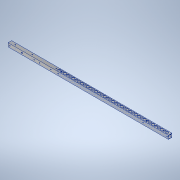
# Autodesk Inventor part: ロボットベース15x15_3
Saved by Autodesk Inventor 2020.3 (Build 243373000, 373)
## iProperties
Created: 2020-07-04
Part Number: ロボットベース15x15_3
Material: アルミニウム 6061
Document SubType Name: Modeling
Designer: totot
Density: 2.7 g/cm^3
Appearance: アルミニウム - フラット
Mass: 98.5001 g
Surface Area: 641.394 cm^2
Volume: 36.4815 cm^3
Author: totot
Autodesk Inventor part; units mm, degrees
ref_plane "YZ Plane" through (0, 0, 0) normal (1, 0, 0) x (0, 1, 0)
ref_plane "XZ Plane" through (0, 0, 0) normal (0, 1, 0) x (-1, 0, 0)
ref_plane "XY Plane" through (0, 0, 0) normal (0, 0, 1) x (1, 0, 0)
sketch "スケッチ1" plane through (0, 0, 0) normal (1, 0, 0) x (0, 1, 0)
  line L0 (0, 0) -> (-15, 0)
  line L1 (-15, 0) -> (-15, 15)
  line L2 (-15, 15) -> (0, 15)
  line L3 (0, 15) -> (0, 0)
  line L4 (-1.2, 13.8) -> (-13.8, 13.8)
  line L5 (-13.8, 13.8) -> (-13.8, 1.2)
  line L6 (-13.8, 1.2) -> (-1.2, 1.2)
  line L7 (-1.2, 1.2) -> (-1.2, 13.8)
  dimension "d0" = 15
  dimension "d1" = 15
  dimension "d2" = 1.2
  dimension "d3" = 1.2
  dimension "d4" = 1.2
  dimension "d5" = 1.2
  constraints: 16 end point, 4 parallel, 2 horizontal, 2 perpendicular
  measures "d0" distance of L1.end L2.end
  measures "d1" distance of L0.end L1.end
  measures "d2" distance between parallel lines of L2 L4
  measures "d3" distance between parallel lines of L7 L3
  measures "d4" distance between parallel lines of L1 L5
  measures "d5" distance between parallel lines of L0 L6
extrude "押し出し1" add sketch "スケッチ1" along normal blind 116
sketch "スケッチ2" plane through (0, -15, 15) normal (0, 0, 1) x (1, 0, 0)
  line L0 (0, 15) -> (116, 15) projected
  line L1 (0, 15) -> (0, 0) projected
  line L2 (116, 15) -> (116, 0) projected
  point P0 (7.5, 7.5)
  point P1 (108.5, 7.5)
  dimension "d8" = 7.5
  dimension "d9" = 7.5
  dimension "d10" = 7.5
  dimension "d11" = 7.5
  measures "d8" distance from line of L0 point (7.5, 7.5)
  measures "d9" distance from line of point (108.5, 7.5) L0
  measures "d10" distance from line of point (7.5, 7.5) L1
  measures "d11" distance from line of point (108.5, 7.5) L2
hole "穴1" at (7.5, -7.5, 15) at (108.5, -7.5, 15) direction (0, 0, -1) diameter 3 end through all
sketch "スケッチ3" plane through (0, -15, 0) normal (0, 0, -1) x (-1, 0, 0)
  circle A0 centre (-7.5, 7.5) radius 1.5 projected
  line L0 (0, 0) -> (-116, 0) projected
  point P0 (0, 15)
  point P1 (-58, 7.5)
  dimension "d19" = 50.5
  dimension "d20" = 7.5
  measures "d19" distance of point (-58, 7.5) A0.centre
  measures "d20" distance from line of point (-58, 7.5) L0
hole "穴2" at (58, -7.5, 0) direction (0, 0, 1) diameter 5 end through all
sketch "スケッチ4" plane through (0, -15, 0) normal (0, -1, 0) x (1, 0, 0)
  line L0 (0, 15) -> (0, 0) projected
  line L1 (0, 0) -> (116, 0) projected
  line L2 (116, 15) -> (116, 0) projected
  point P0 (22.5, 7.5)
  point P1 (93.5, 7.5)
  dimension "d28" = 22.5
  dimension "d29" = 7.5
  dimension "d30" = 7.5
  dimension "d31" = 22.5
  measures "d28" distance from line of point (22.5, 7.5) L0
  measures "d29" distance from line of point (22.5, 7.5) L1
  measures "d30" distance from line of L1 point (93.5, 7.5)
  measures "d31" distance from line of point (93.5, 7.5) L2
hole "穴3" at (22.5, -15, 7.5) at (93.5, -15, 7.5) direction (0, 1, 0) diameter 3 end through all
sketch "スケッチ5" plane through (116, 0, 0) normal (1, 0, 0) x (0, 0, -1)
  line L0 (0, 0) -> (-15, 0)
  line L1 (-15, 0) -> (-15, -15)
  line L2 (-15, -15) -> (0, -15)
  line L3 (0, -15) -> (0, 0)
  line L4 (-13.8, -1.2) -> (-1.2, -1.2) projected
  line L5 (-1.2, -1.2) -> (-13.8, -1.2)
  line L6 (-13.8, -1.2) -> (-13.8, -13.8)
  line L7 (-13.8, -13.8) -> (-1.2, -13.8)
  line L8 (-1.2, -13.8) -> (-1.2, -1.2)
  dimension "d39" = 15
  dimension "d40" = 15
  constraints: 16 end point, 4 parallel, 2 horizontal, 2 perpendicular
  measures "d39" distance of L2.end L1.end
  measures "d40" distance of L1.end L0.end
extrude "押し出し2" add sketch "スケッチ5" along normal blind 99
sketch "スケッチ6" plane through (0, -15, 0) normal (0, 0, -1) x (-1, 0, 0)
  line L0 (-215, 0) -> (-215, 15) projected
  line L1 (0, 15) -> (-215, 15) projected
  point P0 (-207.5, 7.5)
  dimension "d43" = 7.5
  dimension "d44" = 7.5
  measures "d43" distance from line of L0 point (-207.5, 7.5)
  measures "d44" distance from line of L1 point (-207.5, 7.5)
hole "穴4" at (207.5, -7.5, 0) direction (0, 0, 1) diameter 3 end through all
sketch "スケッチ7" plane through (0, 0, 15) normal (0, 1, 0) x (1, 0, 0)
  line L0 (0, 15) -> (215, 15) projected
  line L1 (215, 15) -> (215, 0) projected
  point P0 (192.5, 7.5)
  dimension "d52" = 7.5
  dimension "d53" = 22.5
  measures "d52" distance from line of L0 point (192.5, 7.5)
  measures "d53" distance from line of L1 point (192.5, 7.5)
hole "穴5" at (192.5, 0, 7.5) direction (0, -1, 0) diameter 3 end through all
sketch "スケッチ8" plane through (0, -15, 0) normal (0, 0, -1) x (-1, 0, 0)
  circle A0 centre (-108.5, 7.5) radius 1.5 projected
  line L0 (0, 0) -> (-215, 0) projected
  line L1 (-215, 0) -> (-215, 15) projected
  point P0 (0, 15)
  point P1 (-131, 7.5)
  point P2 (-177.5, 7.5)
  dimension "d61" = 22.5
  dimension "d62" = 7.5
  dimension "d63" = 7.5
  dimension "d64" = 37.5
  measures "d61" distance of point (-131, 7.5) A0.centre
  measures "d62" distance from line of point (-131, 7.5) L0
  measures "d63" distance from line of L0 point (-177.5, 7.5)
  measures "d64" distance from line of L1 point (-177.5, 7.5)
hole "穴6" at (131, -7.5, 0) at (177.5, -7.5, 0) direction (0, 0, 1) diameter 3 end through all
sketch "スケッチ11" plane through (215, 0, 0) normal (1, 0, 0) x (0, 0, -1)
  line L0 (0, -15) -> (0, 0) projected
  line L1 (-15, 0) -> (-15, -15) projected
  line L2 (0, 0) -> (-15, 0)
  line L3 (-15, 0) -> (-15, -15)
  line L4 (-15, -15) -> (0, -15)
  line L5 (0, -15) -> (0, 0)
  line L6 (-1.2, -13.8) -> (-13.8, -13.8) projected
  line L7 (-1.2, -1.2) -> (-13.8, -1.2)
  line L8 (-13.8, -1.2) -> (-13.8, -13.8)
  line L9 (-13.8, -13.8) -> (-1.2, -13.8)
  line L10 (-1.2, -13.8) -> (-1.2, -1.2)
  constraints: 16 end point, 4 parallel, 2 horizontal, 2 perpendicular
extrude "押し出し3" add sketch "スケッチ11" along normal blind 450
sketch "スケッチ12" plane through (0, -15, 0) normal (0, 0, -1) x (-1, 0, 0)
  line L0 (0, 15) -> (-665, 15) projected
  line L1 (-665, 0) -> (-665, 15) projected
  point P0 (-660, 7.5)
  point P1 (-560, 7.5)
  dimension "d114" = 7.5
  dimension "d115" = 5
  dimension "d116" = 7.5
  dimension "d117" = 100
  measures "d114" distance from line of point (-560, 7.5) L0
  measures "d115" distance from line of point (-660, 7.5) L1
  measures "d116" distance from line of point (-660, 7.5) L0
  measures "d117" distance of point (-660, 7.5) point (-560, 7.5)
hole "穴8" at (660, -7.5, 0) at (560, -7.5, 0) direction (0, 0, 1) diameter 3 end through all
sketch "スケッチ13" plane through (0, -15, 0) normal (0, -1, 0) x (1, 0, 0)
  line L0 (0, 15) -> (665, 15) projected
  circle A0 centre (192.5, 7.5) radius 1.5 projected
  line L1 (665, 15) -> (665, 0) projected
  point P0 (0, 0)
  point P1 (653.1875, 7.5)
  point P2 (641.375, 7.5)
  point P3 (629.5625, 7.5)
  point P4 (617.75, 7.5)
  point P5 (605.9375, 7.5)
  point P6 (594.125, 7.5)
  point P7 (582.3125, 7.5)
  point P8 (570.5, 7.5)
  point P9 (558.6875, 7.5)
  point P10 (546.875, 7.5)
  point P11 (535.0625, 7.5)
  point P12 (523.25, 7.5)
  point P13 (511.4375, 7.5)
  point P14 (499.625, 7.5)
  point P15 (487.8125, 7.5)
  point P16 (476, 7.5)
  point P17 (464.1875, 7.5)
  point P18 (452.375, 7.5)
  point P19 (440.5625, 7.5)
  point P20 (428.75, 7.5)
  point P21 (416.9375, 7.5)
  point P22 (405.125, 7.5)
  point P23 (393.3125, 7.5)
  point P24 (381.5, 7.5)
  point P25 (369.6875, 7.5)
  point P26 (357.875, 7.5)
  point P27 (346.0625, 7.5)
  point P28 (334.25, 7.5)
  point P29 (322.4375, 7.5)
  point P30 (310.625, 7.5)
  point P31 (298.8125, 7.5)
  point P32 (287, 7.5)
  point P33 (275.1875, 7.5)
  point P34 (263.375, 7.5)
  point P35 (251.5625, 7.5)
  point P36 (239.75, 7.5)
  point P37 (227.9375, 7.5)
  point P38 (216.125, 7.5)
  point P39 (204.3125, 7.5)
  dimension "d125" = 7.5
  dimension "d126" = 472.5
  dimension "d137" = 11.8125
  dimension "d142" = 11.8125
  constraints: 1 horizontal, 38 other
  measures "d125" distance from line of point (653.188, 7.5) L0
  measures "d126" distance from line of A0.centre L1
  measures "d137" distance of point (653.188, 7.5) point (641.375, 7.5)
  measures "d142" distance from line of point (653.188, 7.5) L1
hole "穴9" at (653.1875, -15, 7.5) at (641.375, -15, 7.5) at (629.5625, -15, 7.5) at (617.75, -15, 7.5) at (605.9375, -15, 7.5) at (594.125, -15, 7.5) at (582.3125, -15, 7.5) at (570.5, -15, 7.5) at (558.6875, -15, 7.5) at (546.875, -15, 7.5) at (535.0625, -15, 7.5) at (523.25, -15, 7.5) at (511.4375, -15, 7.5) at (499.625, -15, 7.5) at (487.8125, -15, 7.5) at (476, -15, 7.5) at (464.1875, -15, 7.5) at (452.375, -15, 7.5) at (440.5625, -15, 7.5) at (428.75, -15, 7.5) at (416.9375, -15, 7.5) at (405.125, -15, 7.5) at (393.3125, -15, 7.5) at (381.5, -15, 7.5) at (369.6875, -15, 7.5) at (357.875, -15, 7.5) at (346.0625, -15, 7.5) at (334.25, -15, 7.5) at (322.4375, -15, 7.5) at (310.625, -15, 7.5) at (298.8125, -15, 7.5) at (287, -15, 7.5) at (275.1875, -15, 7.5) at (263.375, -15, 7.5) at (251.5625, -15, 7.5) at (239.75, -15, 7.5) at (227.9375, -15, 7.5) at (216.125, -15, 7.5) at (204.3125, -15, 7.5) direction (0, 1, 0) diameter 10 end through all
equation "\"d3\" = d2"
equation "\"d4\" = d2"
equation "\"d5\" = d3"
equation "\"d9\" = d8"
equation "\"d10\" = d8"
equation "\"d11\" = d9"
equation "\"d30\" = d29"
equation "\"d31\" = d28"
equation "\"d63\" = d62"
equation "\"d116\" = d114"
equation "\"d137\" = 0.025 * d126"
equation "\"d142\" = d137"
